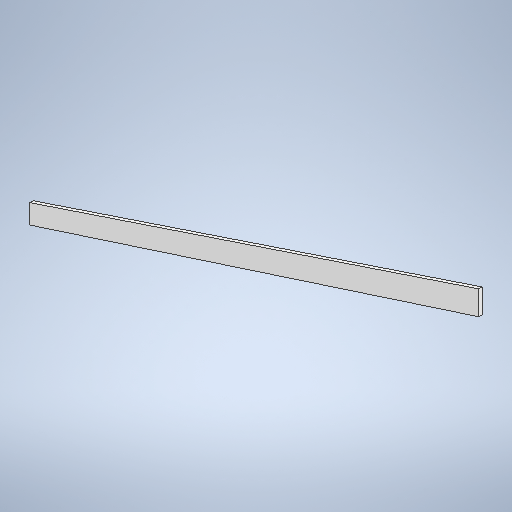
# Autodesk Inventor part: Fascia_For_Side
Saved by Autodesk Inventor 2025.1 (Build 291241020, 241B)
## iProperties
Created: 2024-09-15
Part Number: Fascia_For_Side
Material: Generic
Document SubType Name: Modeling
Designer: Tom
Density: 1 g/cm^3
Appearance: White
Author: Tom
Autodesk Inventor part; units mm, degrees
ref_plane "XZ Plane" through (0, 0, 0) normal (0, 1, 0) x (-1, 0, 0)
ref_plane "XY Plane" through (0, 0, 0) normal (0, 0, 1) x (1, 0, 0)
sketch "Sketch1" plane through (0, 0, 0) normal (0, 0, 1) x (1, 0, 0)
  line L0 (0, 0) -> (3295.8151, 1099.6737)
  line L1 (3295.8151, 1246.9448) -> (-135.0962, 102.1952)
  line L2 (0, 0) -> (-135.0962, 0)
  line L3 (-135.0962, 0) -> (-135.0962, 102.1952)
  line L4 (-135.0962, 102.1952) -> (1593.1098, 678.8242)
  line L5 (3295.8151, 1099.6737) -> (3263.9, 1099.6737)
  line L6 (3295.8151, 1099.6737) -> (3295.8151, 1246.9448)
  line L7 (-88.9, 0) -> (-88.9, 117.6089)
  line L8 (3263.9, 1089.025) -> (3263.9, 1236.2961)
  line L9 (-135.0962, 102.1952) -> (-135.0962, -46.09)
  line L10 (-135.0962, -46.09) -> (3295.8151, 1062.5408)
  line L11 (3295.8151, 1062.5408) -> (3295.8151, 1099.6737)
  dimension "d5" = 139.7
  dimension "d17" = 88.9
  dimension "d19" = 3352.8
  dimension "d23" = 31.9151
  dimension "d28" = 46.1962
  dimension "d33" = 1089.025
  dimension "d36" = 148.2852
  dimension "d37" = 184.404
  constraints: 24 end point, 5 point on line, 5 vertical, 2 coincident, 2 collinear, 2 horizontal
  measures "d5" distance between parallel lines of L1 L0
  measures "d17" distance from line of L7 point (0, 0)
  measures "d19" distance between parallel lines of L7 L8
  measures "d23" distance between parallel lines of L6 L8
  measures "d28" distance between parallel lines of L3 L7
  measures "d33" vertical distance of L8.start point (0, 0)
  measures "d36" distance of L1.end L9.end
  measures "d37" distance of L1.start L10.end
extrude "Extrusion2" add sketch "Sketch1" along normal blind 25.4
ref_plane "Work Plane2" through (-135.0962, -46.09, 0) normal (0, 1, 0) x (0, 0, 1)
body "Solid2"
